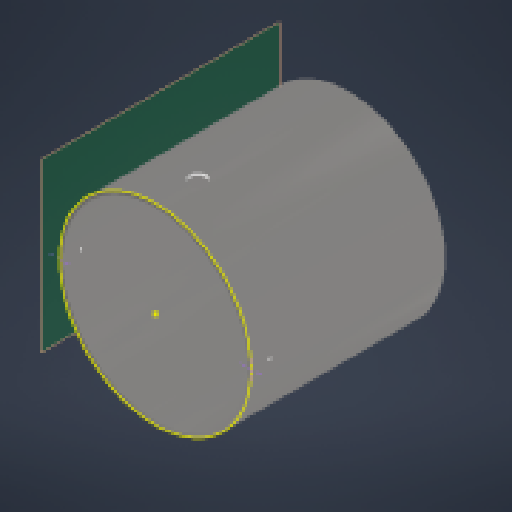
# Autodesk Inventor part: Electromagnetic cover body
Saved by Autodesk Inventor 2026.3 (Build 303398000, 398)
## iProperties
Created: 2026-08-03
Part Number: Electromagnetic cover body
Material: Generic
Document SubType Name: Sheet Metal
Designer: matot
Density: 1 g/cm^3
Sheet Metal Rule: Default_mm
Appearance: Default
Author: matot
Autodesk Inventor part; units mm, degrees
ref_plane "YZ Plane" through (0, 0, 0) normal (1, 0, 0) x (0, 1, 0)
ref_plane "XZ Plane" through (0, 0, 0) normal (0, 1, 0) x (-1, 0, 0)
ref_plane "XY Plane" through (0, 0, 0) normal (0, 0, 1) x (1, 0, 0)
sketch "Sketch1" plane through (0, 0, 0) normal (0, 0, 1) x (1, 0, 0)
  circle A0 centre (0, 0) radius 57
  circle A1 centre (0, 0) radius 55
  dimension "d0" = 114
  dimension "d1" = 110
  constraints: 2 centre point, 2 coincident
  measures "d0" diameter of A0
  measures "d1" diameter of A1
extrude "Extrusion1" add sketch "Sketch1" along normal blind 115
sketch "Sketch2" plane through (0, 0, 115) normal (0, 0, 1) x (1, 0, 0)
  circle A0 centre (0, 0) radius 57 projected
  point P0 (0, 57)
  constraints: 1 vertical alignment, 1 other
ref_plane "Work Plane1" through (0, 57, 115) normal (0, 1, 0) x (-1, 0, 0)
sketch "Sketch3" plane through (0, 57, 115) normal (0, 1, 0) x (-1, 0, 0)
  line L0 (57, 0) -> (-57, 0) projected
  point P0 (0, -115)
  point P1 (0, -25)
  dimension "d4" = 25
  measures "d4" distance from line of L0 point (0, -25)
hole "Hole1" at (0, 57, 90) direction (0, -1, 0) diameter 10 depth 20 tip angle 118
sketch "Sketch4" plane through (0, 0, 115) normal (0, 0, 1) x (1, 0, 0)
  circle A0 centre (0, 0) radius 57 projected
  point P0 (-57, 0)
  point P1 (57, 0)
  constraints: 1 horizontal alignment, 1 other
ref_plane "Work Plane3" through (-57, 0, 115) normal (-1, 0, 0) x (0, -1, 0)
sketch "Sketch5" plane through (-57, 0, 115) normal (-1, 0, 0) x (0, -1, 0)
  line L0 (57, 0) -> (-57, 0) projected
  point P0 (0, -115)
  point P1 (0, -11)
  dimension "d12" = 11
  measures "d12" distance from line of L0 point (0, -11)
hole "Hole2" at (-57, 0, 104) direction (1, 0, 0) diameter 2 end through all
equation "\"d18\" = Thickness"
equation "\"BendRadius\" = Thickness"
equation "\"BendReliefWidth\" = Thickness"
equation "\"BendReliefDepth\" = 0.5 * Thickness"
equation "\"CornerReliefSize\" = 4 * Thickness"
equation "\"MinimumRemnant\" = 2 * Thickness"
equation "\"TransitionRadius\" = BendRadius"
equation "\"JacobiRadiusSize\" = BendRadius"
equation "\"GapSize\" = Thickness"
equation "\"Thickness\" = 0.5"
body "Solid1"
